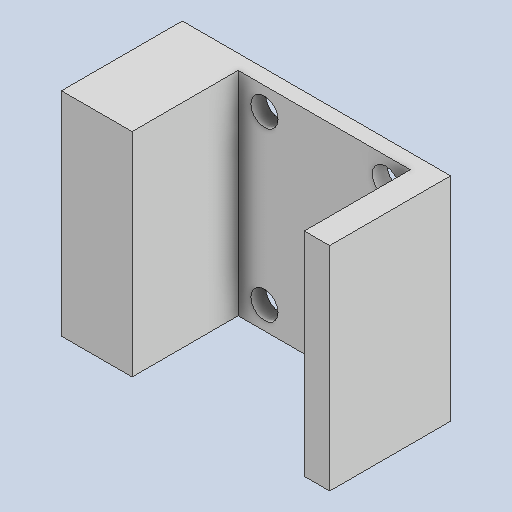
# Autodesk Inventor part: DriverCC
Saved by Autodesk Inventor 2023 (Build 270158000, 158)
## iProperties
Created: 2023-01-01
Part Number: DriverCC
Material: Genérico
Document SubType Name: Modeling
Designer: sergi
Density: 1 g/cm^3
Appearance: Valor por defecto
Author: sergi
Autodesk Inventor part; units mm, degrees
ref_plane "YZ Plane" through (0, 0, 0) normal (1, 0, 0) x (0, 1, 0)
ref_plane "Plano de trabajo2" through (0.003, 0, 0) normal (0, 0, 1) x (1, 0.0001, 0)
sketch "Boceto1" plane through (0.003, 0, 0) normal (0, 0, 1) x (1, 0.0001, 0)
  line L0 (-0.003, 0) -> (29.597, 0)
  line L1 (29.597, 0) -> (29.597, 23.45)
  line L2 (29.597, 23.45) -> (-0.003, 23.45)
  line L3 (-0.003, 23.45) -> (-0.003, 0)
  line L4 (29.597, 0) -> (29.597, 4)
  line L5 (29.597, 23.45) -> (29.597, 19.45)
  circle A0 centre (24.097, 20.95) radius 1.5
  circle A1 centre (24.097, 2.5) radius 1.5
  circle A2 centre (10.697, 20.95) radius 1.5
  circle A3 centre (10.697, 2.5) radius 1.5
  dimension "d0" = 29.6
  dimension "d1" = 23.45
  dimension "d5" = 3
  dimension "d6" = 3
  dimension "d16" = 3
  dimension "d17" = 3
  constraints: 12 end point, 4 centre point, 2 parallel, 2 point on line, 1 horizontal, 1 perpendicular
  measures "d0" distance of L2.end L1.end
  measures "d1" distance of L1.end L0.end
  measures "d5" diameter of A0
  measures "d6" diameter of A1
  measures "d16" diameter of A2
  measures "d17" diameter of A3
extrude "Extrusión1" add sketch "Boceto1" along normal blind 1.64
ref_plane "Plano de trabajo4" through (0.003, 0, 1.64) normal (0, 0, 1) x (1, 0.0001, 0)
sketch "Boceto2" plane through (0.003, 0, 1.64) normal (0, 0, 1) x (1, 0.0001, 0)
  line L0 (29.597, 0) -> (29.597, 23.45) projected
  line L1 (-0.003, 0) -> (29.597, 0) projected
  line L2 (29.597, 23.45) -> (26.797, 23.45)
  line L3 (26.797, 23.45) -> (26.797, 0)
  line L4 (26.797, 0) -> (29.597, 0)
  line L5 (29.597, 0) -> (29.597, 23.45)
  line L6 (-0.003, 0) -> (7.797, 0)
  line L7 (7.797, 0) -> (7.797, 23.45)
  line L8 (7.797, 23.45) -> (-0.003, 23.45)
  line L9 (-0.003, 23.45) -> (-0.003, 0)
  point P0 (7.797, 0)
  dimension "d12" = 2.8
  dimension "d13" = 7.8
  constraints: 16 end point, 4 parallel, 2 horizontal, 2 perpendicular, 2 point on line
  measures "d12" distance of L4.end L3.end
  measures "d13" distance of L8.end L7.end
extrude "Extrusión2" add sketch "Boceto2" along normal blind 11.7
